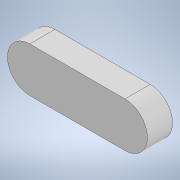
# Autodesk Inventor part: key5
Saved by Autodesk Inventor 2020 (Build 240168000, 168)
## iProperties
Created: 2021-06-15
Part Number: key5
Material: 常规
Document SubType Name: Modeling
Designer: dell
Density: 1 g/cm^3
Appearance: 默认
Author: dell
Autodesk Inventor part; units mm, degrees
ref_plane "YZ Plane" through (0, 0, 0) normal (1, 0, 0) x (0, 1, 0)
ref_plane "XZ Plane" through (0, 0, 0) normal (0, 1, 0) x (-1, 0, 0)
ref_plane "XY Plane" through (0, 0, 0) normal (0, 0, 1) x (1, 0, 0)
sketch "草图1" plane through (0, 0, 0) normal (0, 0, 1) x (1, 0, 0)
  line L0 (-34, 0) -> (34, 0) construction
  line L1 (-34, -16) -> (34, -16)
  line L2 (34, 16) -> (-34, 16)
  arc A0 (-34, 16) -> (-34, -16) centre (-34, 0) ccw
  arc A1 (34, -16) -> (34, 16) centre (34, 0) ccw
  line L3 (-70, 0) -> (70, 0) construction
  line L4 (0, 22.4) -> (0, -22.4) construction
  point P0 (0, 0)
  dimension "d2" = 100
  dimension "d3" = 32
  constraints: 8 end point, 4 point on circle, 4 tangent, 2 centre point, 1 horizontal, 1 midpoint, 1 parallel, 1 symmetric about line, 1 other
  measures "d3" distance between parallel lines of L1 L2
extrude "拉伸2" add sketch "草图1" along normal blind 18
